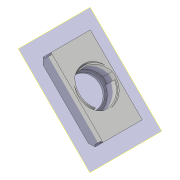
# Autodesk Inventor part: 20_Cube_Insert_Mirror_Holder_v2
Saved by Autodesk Inventor 2019 (Build 230136000, 136)
## iProperties
Created: 2019-07-22
Part Number: 20_Cube_Insert_Mirror_Holder_v2
Material: Generic
Document SubType Name: Modeling
Designer: diederichbenedict
Density: 1 g/cm^3
Appearance: Default
Author: diederichbenedict
Autodesk Inventor part; units mm, degrees
ref_plane "YZ Plane" through (0, 0, 0) normal (1, 0, 0) x (0, 1, 0)
ref_plane "XZ Plane" through (0, 0, 0) normal (0, 1, 0) x (-1, 0, 0)
ref_plane "XY Plane" through (0, 0, 0) normal (0, 0, 1) x (1, 0, 0)
sketch "Sketch1" plane through (0, 0, 0) normal (0, 0, 1) x (1, 0, 0)
  line L0 (-16.9, 21.4) -> (-16.9, 16.9) construction
  arc A0 (-22.9, 19.9) -> (-19.9, 22.9) centre (-19.9, 19.9) ccw construction
  line L1 (-16.9, 16.9) -> (16.9, 16.9) construction
  line L2 (16.9, 16.9) -> (16.9, -16.9) construction
  line L3 (16.9, -16.9) -> (-16.9, -16.9) construction
  line L4 (-16.9, -16.9) -> (-16.9, 16.9) construction
  arc A1 (22.9, -19.9) -> (19.9, -22.9) centre (19.9, -19.9) ccw construction
  line L5 (22.9, 19.9) -> (22.9, -19.9) construction
  arc A2 (19.9, 22.9) -> (22.9, 19.9) centre (19.9, 19.9) ccw construction
  line L6 (-19.9, 22.9) -> (19.9, 22.9) construction
  arc A3 (-22.9, 19.9) -> (-19.9, 22.9) centre (-19.9, 19.9) ccw construction
  line L7 (-22.9, -19.9) -> (-22.9, 19.9) construction
  arc A4 (-19.9, -22.9) -> (-22.9, -19.9) centre (-19.9, -19.9) ccw construction
  line L8 (19.9, -22.9) -> (-19.9, -22.9) construction
  line L9 (-21.4, 16.9) -> (-16.9, 16.9) construction
  line L10 (-16.9, -16.9) -> (-21.4, -16.9) construction
  line L11 (-16.9, -16.9) -> (-16.9, -21.4) construction
  line L12 (16.9, -21.4) -> (16.9, -16.9) construction
  line L13 (21.4, -16.9) -> (16.9, -16.9) construction
  line L14 (16.9, 16.9) -> (21.4, 16.9) construction
  line L15 (16.9, 16.9) -> (16.9, 21.4) construction
  line L16 (-16.8009, 21.2415) -> (21.2415, -16.8009)
  line L17 (21.2415, -16.8009) -> (16.8009, -21.2415)
  line L18 (16.8009, -21.2415) -> (-21.2415, 16.8009)
  line L19 (-21.2415, 16.8009) -> (-16.8009, 21.2415)
  line L20 (-16.8009, 21.2415) -> (16.8009, -21.2415) construction
  line L21 (21.2415, -16.8009) -> (-21.2415, 16.8009) construction
  line L22 (-16.8009, 21.2415) -> (36.9991, 21.2415) construction
  line L23 (-21.2415, 16.8009) -> (-22.9, 16.8009)
  line L24 (16.8009, -21.2415) -> (16.8009, -22.9)
  line L25 (16.8009, -22.9) -> (-22.9, 16.8009)
  line L26 (-16.8009, 21.2415) -> (-16.8009, 22.9)
  line L27 (21.2415, -16.8009) -> (22.9, -16.8009)
  line L28 (22.9, -16.8009) -> (-16.8009, 22.9)
  line L29 (-22.9, 16.8009) -> (-22.9, 11.5863)
  line L30 (16.8009, -22.9) -> (11.5863, -22.9)
  line L31 (-22.9, 11.5863) -> (11.5863, -22.9)
  point P0 (0, 0)
  dimension "d0" = 53.8
  dimension "d1" = 45
  dimension "d2" = 6.28
  dimension "d5" = 8
  constraints: 32 end point, 6 point on line, 4 parallel, 4 perpendicular, 2 midpoint, 1 equal length, 1 horizontal
  measures "d0" distance of L16.start L16.end
  measures "d1" angle of L16 L22
  measures "d2" distance of L16.end L17.end
  measures "d5" distance from line of L31 point (0, 0)
extrude "Extrusion1" add sketch "Sketch1" along normal blind 30
ref_plane "Work Plane1" through (16.9, -16.9, -8) normal (-0.7071, -0.7071, 0) x (0, 0, 1)
sketch "Sketch2" plane through (16.9, -16.9, -8) normal (-0.7071, -0.7071, 0) x (0, 0, 1)
  line L0 (8, -4.1725) -> (8, 51.973) projected
  line L1 (8, 51.973) -> (38, 51.973) projected
  line L2 (38, -4.1725) -> (38, 51.973) projected
  line L3 (8, -4.1725) -> (38, -4.1725) projected
  circle A0 centre (23, 23.9002) radius 14
  point P0 (8, 23.9002)
  dimension "d6" = 28
  dimension "d13" = 15
  constraints: 1 centre point
  measures "d6" diameter of A0
  measures "d13" distance from line of A0.centre L0
extrude "Extrusion2" cut sketch "Sketch2" along normal blind 6 and the other way blind 6 contours A0
sketch "Sketch3" plane through (-4.2426, -4.2426, 15) normal (0.7071, 0.7071, 0) x (-0.7071, 0.7071, 0)
  circle A0 centre (0, 0) radius 14 projected
  circle A1 centre (0, 0) radius 11.119
  point P0 (0, -15)
  constraints: 1 centre point
extrude "Extrusion3" cut sketch "Sketch3" against normal blind 6 contours A1
sketch "Sketch4" plane through (-16.8009, 22.9, 0) normal (0.7071, 0.7071, 0) x (-0.7071, 0.7071, 0)
  circle A0 centre (-28.0727, 15) radius 14 projected
  arc A1 (-20.2691, 3.3766) -> (-15.8567, 19.6091) centre (-30.0482, 14.7507) ccw
  arc A2 (-25.4219, 1.2532) -> (-16.3567, 19.6091) centre (-30.7204, 15.2863) ccw
  line L0 (-15.8567, 19.6091) -> (-16.3567, 19.6091)
  line L1 (-56.1455, 30) -> (0, 30) projected
  arc A3 (-25.4219, 1.2532) -> (-20.2691, 3.3766) centre (-28.0727, 15) ccw
  point P0 (-28.0727, 0)
  dimension "d14" = 0.5
  dimension "d15" = 15
  dimension "d16" = 15
  constraints: 8 point on circle, 3 centre point, 2 end point, 1 concentric, 1 parallel
  measures "d14" distance of L0.end L0.start
  measures "d15" radius of A1
  measures "d16" radius of A2
extrude "Extrusion4" add sketch "Sketch4" against normal blind 10 contours A2 L0 A1 A0 picked at (-18.6617, 5.9923)
pattern_circular "Circular Pattern1" count 3 over 360 about axis through (0, 0, 15) along (-0.7071, -0.7071, 0) of "Extrusion4"
equation "\"d3\" = MirrorThickness1"
equation "\"d13\" = 0.5 * MirrorThickness1"
equation "\"MirrorThickness1\" = 30"
body "Solid1"
